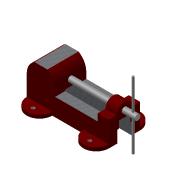
# Autodesk Inventor part: Vise_Substitute
Saved by Autodesk Inventor 2022 (Build 260148000, 148)
## iProperties
Created: 2006-01-18
Part Number: Vise_Substitute
Document SubType Name: Modeling
Designer: PMiller
Material: Cast Steel
Density: 7.85 g/cm^3
Appearance: Red (Cast)
Author: PMiller
Autodesk Inventor part; units mm, degrees
note: some values were not read from the file. Chosen so that the rebuilt part matches the saved one: direction of "Hole1".
ref_plane "YZ Plane" through (0, 0, 0) normal (1, 0, 0) x (0, 1, 0)
sketch "Sketch1" plane through (0, 0, 0) normal (0, 0, 1) x (1, 0, 0)
  line L0 (-63.5, -31.75) -> (-63.5, -23.8125)
  line L1 (-63.5, -23.8125) -> (-34.925, -23.8125)
  line L2 (-34.925, -23.8125) -> (-34.925, 23.8125)
  line L3 (-34.925, 23.8125) -> (-17.4625, 23.8125)
  arc A0 (17.4625, 23.8125) -> (-17.4625, 23.8125) centre (0, 23.8125) ccw
  line L4 (17.4625, 23.8125) -> (34.925, 23.8125)
  line L5 (34.925, 23.8125) -> (34.925, -23.8125)
  line L6 (34.925, -23.8125) -> (63.5, -23.8125)
  line L7 (63.5, -23.8125) -> (63.5, -31.75)
  line L8 (63.5, -31.75) -> (-63.5, -31.75)
  point P0 (0, 0)
  point P1 (-34.925, 0)
  dimension "d0" = 28.575
  dimension "d1" = 55.5625
  dimension "d2" = 17.4625
  dimension "d3" = 7.9375
  dimension "d4" = 69.85
  constraints: 18 end point, 6 parallel, 4 equal length, 2 point on circle, 1 centre point, 1 collinear, 1 horizontal alignment, 1 midpoint, 1 perpendicular, 1 point on line, 1 vertical, 1 vertical alignment
  measures "d0" distance of L0.end L1.end
  measures "d1" distance between parallel lines of L3 L8
  measures "d2" radius of A0
  measures "d3" distance of L0.start L0.end
  measures "d4" distance between parallel lines of L5 L2
extrude "Extrusion1" add sketch "Sketch1" along normal blind 184.15
sketch "Sketch2" plane through (-63.5, -23.8125, 0) normal (0, 1, 0) x (1, 0, 0)
  line L0 (0, -184.15) -> (28.575, -184.15) projected
  line L1 (28.575, 0) -> (28.575, -184.15) projected
  line L2 (0, 0) -> (28.575, 0) projected
  line L3 (0, 0) -> (0, -184.15) projected
  line L4 (0, -57.15) -> (28.575, -57.15)
  line L5 (0, -127) -> (28.575, -127)
  dimension "d7" = 57.15
  dimension "d8" = 57.15
  constraints: 4 end point, 4 point on line, 1 parallel, 1 perpendicular
  measures "d7" distance between parallel lines of L0 L5
  measures "d8" distance between parallel lines of L2 L4
extrude "Extrusion2" cut sketch "Sketch2" against normal through all contours L3 L4 L1 L5
mirror "Mirror1" about plane through (0, 0, 0) normal (1, 0, 0) of "Extrusion2"
sketch "Sketch3" plane through (-34.925, -23.8125, 0) normal (-1, 0, 0) x (0, 0, 1)
  line L0 (0, 0) -> (0, 47.625)
  line L1 (127, -7.9375) -> (57.15, -7.9375)
  line L2 (0, 65.0875) -> (184.15, 65.0875)
  line L3 (0, 65.0875) -> (0, 47.625)
  line L4 (0, 31.75) -> (158.75, 31.75)
  line L5 (158.75, 31.75) -> (158.75, 65.0875)
  line L6 (184.15, 0) -> (184.15, 47.625) projected
  line L7 (0, 47.625) -> (184.15, 47.625) projected
  line L8 (0, 0) -> (0, 47.625) projected
  line L9 (0, 0) -> (57.15, 0) projected
  line L10 (57.15, 0) -> (57.15, -7.9375) projected
  line L11 (127, -7.9375) -> (57.15, -7.9375) projected
  line L12 (127, 0) -> (127, -7.9375) projected
  line L13 (127, 0) -> (184.15, 0) projected
  dimension "d11" = 39.6875
  dimension "d12" = 158.75
  constraints: 12 end point, 2 perpendicular, 2 point on line
  measures "d11" distance between parallel lines of L1 L4
  measures "d12" distance between parallel lines of L5 L0
extrude "Extrusion3" cut sketch "Sketch3" against normal through all contours L0 L7 L5 L4 | L3 L2 L5 L7
sketch "Sketch4" plane through (-34.925, -23.8125, 184.15) normal (-1, 0, 0) x (0, 0, 1)
  line L0 (-25.4, 31.75) -> (-184.15, 31.75) projected
  line L1 (-25.4, 47.625) -> (-25.4, 31.75) projected
  line L2 (-184.15, 31.75) -> (-184.15, 46.0375)
  arc A0 (-152.4, 80.8179) -> (-184.15, 46.0375) centre (-149.225, 46.0375) ccw
  line L3 (-166.8312, 76.2) -> (-152.4, 76.2)
  line L4 (-152.4, 76.2) -> (-152.4, 31.75)
  line L5 (-25.4, 47.625) -> (0, 47.625) projected
  line L6 (-152.4, 76.2) -> (-152.4, 80.8179)
  line L7 (-120.65, 31.75) -> (-120.65, 46.0375)
  arc A1 (-120.65, 46.0375) -> (-152.4, 80.8179) centre (-155.575, 46.0375) ccw
  line L8 (-137.9688, 76.2) -> (-152.4, 76.2)
  line L9 (-152.4, 31.75) -> (-120.65, 31.75)
  dimension "d15" = 31.75
  dimension "d16" = 34.925
  dimension "d17" = 44.45
  dimension "d18" = 30.1625
  constraints: 14 end point, 6 point on circle, 4 symmetric about line, 2 centre point, 2 parallel, 2 perpendicular, 1 collinear, 1 point on line, 1 tangent, 1 other
  measures "d15" distance between parallel lines of L4 L2
  measures "d16" radius of A0
  measures "d17" distance between parallel lines of L0 L3
  measures "d18" distance from line of L3 A0.centre
extrude "Extrusion4" add sketch "Sketch4" against normal up to surface (69.85 mm away) contours L0 L4 L8 A1 L7 | L0 L2 A0 L3 L4
sketch "Sketch5" plane through (0, 0, 184.15) normal (0, 0, 1) x (1, 0, 0)
  line L0 (63.5, -31.75) -> (-63.5, -31.75) projected
  arc A0 (17.4625, 23.8125) -> (-17.4625, 23.8125) centre (0, 23.8125) ccw projected
  line L1 (-34.925, -23.8125) -> (-34.925, 23.8125) projected
  line L2 (-15.875, -31.75) -> (-15.875, -4.7625)
  line L3 (-15.875, -4.7625) -> (-12.7, -4.7625)
  line L4 (-12.7, -4.7625) -> (-12.7, 11.1125)
  line L5 (-12.7, 11.1125) -> (12.7, 11.1125)
  line L6 (12.7, 11.1125) -> (12.7, -4.7625)
  line L7 (12.7, -4.7625) -> (15.875, -4.7625)
  line L8 (15.875, -4.7625) -> (15.875, -31.75)
  point P0 (0, 11.1125)
  dimension "d22" = 31.75
  dimension "d23" = 25.4
  dimension "d24" = 26.9875
  dimension "d25" = 42.8625
  constraints: 14 end point, 4 parallel, 2 equal length, 2 perpendicular, 2 point on line, 1 collinear, 1 midpoint, 1 vertical alignment
  measures "d22" distance between parallel lines of L8 L2
  measures "d23" distance between parallel lines of L6 L4
  measures "d24" distance of L7.end L8.end
  measures "d25" distance between parallel lines of L0 L5
extrude "Extrusion5" cut sketch "Sketch5" against normal through all
fillet "Fillet1" radius 28.575 8 edges at (-63.5, -27.7812, 0) (-63.5, -27.7812, 57.15) (-63.5, -27.7812, 127) (-63.5, -27.7812, 184.15) (63.5, -27.7812, 184.15) (63.5, -27.7812, 127) (63.5, -27.7812, 57.15) (63.5, -27.7812, 0)
sketch "Sketch8" plane through (0, 0, 184.15) normal (0, 0, 1) x (1, 0, 0)
  line L0 (-15.875, -31.75) -> (-34.925, -31.75) projected
  arc A0 (17.4625, 23.8125) -> (-17.4625, 23.8125) centre (0, 23.8125) ccw projected
  point P0 (0, 25.4)
  dimension "d59" = 57.15
  constraints: 1 vertical alignment
  measures "d59" distance from line of point (0, 25.4) L0
hole "Hole1" at (0, 25.4, 184.15) direction (0, 0, -1) diameter 12.7 end up to surface thread size "5/8-8 Acme" class "2G" standard "ACME"
sketch "Sketch7" plane through (-34.925, -23.8125, 57.15) normal (0, 1, 0) x (1, 0, 0)
  line L0 (0, 57.15) -> (0, 0) projected
  point P0 (-14.2875, 28.575)
  point P1 (0, 28.575)
  dimension "d47" = 14.2875
  constraints: 1 horizontal alignment, 1 midpoint
  measures "d47" distance from line of L0 point (-14.287, 28.575)
hole "Hole3" at (-49.2125, -23.8125, 28.575) direction (0, -1, 0) diameter 7.9375 end through all
ref_plane "Work Plane1" through (0, 0, 92.075) normal (0, 0, 1) x (1, 0, 0)
mirror "Mirror2" about plane through (0, 0, 92.075) normal (0, 0, 1) of "Hole3"
mirror "Mirror3" about plane through (0, 0, 0) normal (1, 0, 0) of "Hole3", "Mirror2"
sketch "Sketch9" plane through (-34.925, 7.9375, 63.5) normal (0, 0, 1) x (1, 0, 0)
  circle A0 centre (34.925, 17.4625) radius 6.35 projected
extrude "Extrusion6" add sketch "Sketch9" along normal blind 150
ref_plane "Work Plane2" through (0, 25.4, 63.5) normal (0, 1, 0) x (0, 0, 1)
sketch "Sketch10" plane through (0, 25.4, 63.5) normal (0, 1, 0) x (0, 0, 1)
  circle A0 centre (140, 0) radius 2.5229
  line L0 (150, 6.35) -> (150, -6.35) projected
  point P0 (150, 0)
  dimension "d63" = 10
  constraints: 1 centre point, 1 horizontal alignment, 1 midpoint
  measures "d63" distance from line of L0 A0.centre
extrude "Extrusion7" add sketch "Sketch10" along normal mid plane 150
equation "\"d7\" = 2 * d0"
equation "\"d8\" = 2 * d0"
equation "\"d47\" = 0.5 * d0"
body "Solid1"
